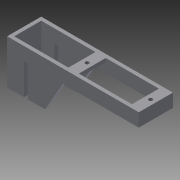
# Autodesk Inventor part: CarCab
Saved by Autodesk Inventor 2015 (Build 190159000, 159)
## iProperties
Created: 2016-04-06
Part Number: CarCab
Material: Generic
Document SubType Name: Modeling
Designer: Lee
Density: 1 g/cm^3
Appearance: Default
Author: Lee
Autodesk Inventor part; units mm, degrees
ref_plane "YZ Plane" through (0, 0, 0) normal (1, 0, 0) x (0, 1, 0)
ref_plane "XZ Plane" through (0, 0, 0) normal (0, 1, 0) x (-1, 0, 0)
ref_plane "XY Plane" through (0, 0, 0) normal (0, 0, 1) x (1, 0, 0)
sketch "Sketch1" plane through (0, 0, 0) normal (0, 0, 1) x (1, 0, 0)
  line L0 (0, 0) -> (59.5, 0)
  line L1 (59.5, 0) -> (59.5, 15.4)
  line L2 (59.5, 15.4) -> (0, 15.4)
  line L3 (0, 15.4) -> (0, 0)
  line L4 (1.6, 13.8) -> (57.9, 13.8)
  line L5 (57.9, 13.8) -> (57.9, 1.6)
  line L6 (57.9, 1.6) -> (1.6, 1.6)
  line L7 (1.6, 1.6) -> (1.6, 13.8)
  dimension "d0" = 59.5
  dimension "d1" = 15.4
  dimension "d2" = 1.6
  constraints: 16 end point, 4 parallel, 2 perpendicular, 1 horizontal, 3 other
  measures "d0" distance of L1.end L2.end
  measures "d1" distance of L2.end L0.start
  measures "d2" distance between parallel lines of L2 L4
extrude "Extrusion1" add sketch "Sketch1" along normal blind 20
sketch "Sketch2" plane through (0, 0, 0) normal (0, -1, 0) x (1, 0, 0)
  line L0 (1.6, 0) -> (57.9, 0) projected
  line L1 (7.6, 0) -> (9.2, 0)
  line L2 (9.2, 0) -> (9.2, 14)
  line L3 (9.2, 14) -> (7.6, 14)
  line L4 (7.6, 14) -> (7.6, 0)
  line L5 (0, 0) -> (0, 20) projected
  dimension "d5" = 1.6
  dimension "d6" = 14
  dimension "d7" = 7.6
  constraints: 8 end point, 2 parallel, 1 horizontal, 1 perpendicular, 1 point on line
  measures "d5" distance of L2.end L3.end
  measures "d6" distance of L1.end L2.end
  measures "d7" distance between parallel lines of L5 L4
extrude "Extrusion2" cut sketch "Sketch2" against normal up to surface (15.4 mm away)
sketch "Sketch3" plane through (0, 0, 20) normal (0, -1, 0) x (1, 0, 0)
  line L0 (9.2, -6) -> (9.2, -20) projected
  line L1 (9.2, -20) -> (59.5, -20) projected
  line L2 (59.5, -20) -> (59.5, 0) projected
  line L3 (0, 0) -> (59.5, 0) projected
  line L4 (0, -20) -> (0, 0) projected
  line L5 (0, -20) -> (7.6, -20) projected
  line L6 (7.6, -20) -> (7.6, -6) projected
  line L7 (7.6, -6) -> (9.2, -6) projected
  line L8 (57.9, -20) -> (9.2, -20) projected
  line L9 (25.2, -20) -> (59.5, -20)
  line L10 (59.5, -20) -> (59.5, -6)
  line L11 (59.5, -6) -> (25.2, -6)
  line L12 (25.2, -6) -> (25.2, -20)
  dimension "d10" = 14
  dimension "d11" = 16
  constraints: 8 end point, 2 parallel, 2 point on line, 1 horizontal, 1 perpendicular
  measures "d10" distance of L11.end L9.start
  measures "d11" distance between parallel lines of L0 L12
extrude "Extrusion3" cut sketch "Sketch3" against normal up to surface (15.4 mm away) contours L12 L11 L2 L1
sketch "Sketch4" plane through (0, 0, 20) normal (0, -1, 0) x (1, 0, 0)
  line L0 (25.2, -6) -> (59.5, -6) projected
  line L1 (59.5, -6) -> (59.5, 0) projected
  line L2 (0, 0) -> (59.5, 0) projected
  line L3 (0, -20) -> (0, 0) projected
  line L4 (0, -20) -> (7.6, -20) projected
  line L5 (7.6, -20) -> (7.6, -6) projected
  line L6 (7.6, -6) -> (9.2, -6) projected
  line L7 (9.2, -6) -> (9.2, -20) projected
  line L8 (9.2, -20) -> (25.2, -20) projected
  line L9 (25.2, -20) -> (25.2, -6) projected
  line L10 (59.5, 0) -> (54.8, 0)
  line L11 (54.8, 0) -> (54.8, -1.6)
  line L12 (54.8, -1.6) -> (59.5, -1.6)
  line L13 (59.5, -1.6) -> (59.5, 0)
  line L14 (57.9, 0) -> (1.6, 0) projected
  line L15 (30.8, 0) -> (26.1, 0)
  line L16 (26.1, 0) -> (26.1, -1.6)
  line L17 (26.1, -1.6) -> (30.8, -1.6)
  line L18 (30.8, -1.6) -> (30.8, 0)
  dimension "d14" = 4.7
  dimension "d15" = 1.6
  dimension "d16" = 1.6
  dimension "d17" = 4.7
  dimension "d18" = 24
  constraints: 16 end point, 4 parallel, 2 horizontal, 2 perpendicular, 1 point on line
  measures "d14" distance of L11.end L12.end
  measures "d15" distance of L10.end L11.end
  measures "d16" distance of L15.end L16.end
  measures "d17" distance of L16.end L17.end
  measures "d18" distance between parallel lines of L11 L18
extrude "Extrusion4" add sketch "Sketch4" against normal up to next contours L12 L11 L2 L1 | L18 L17 L16 L2
sketch "Sketch6" plane through (0, 0, 20) normal (0, 0, 1) x (1, 0, 0)
  line L0 (0, 0) -> (59.5, 0) projected
  line L1 (59.5, 0) -> (59.5, 15.4) projected
  line L2 (59.5, 15.4) -> (0, 15.4) projected
  line L3 (0, 15.4) -> (0, 0) projected
  line L4 (26.1, 1.6) -> (26.1, 13.8) projected
  line L5 (26.1, 1.6) -> (1.6, 1.6) projected
  line L6 (1.6, 1.6) -> (1.6, 13.8) projected
  line L7 (1.6, 13.8) -> (26.1, 13.8) projected
  line L8 (54.8, 1.6) -> (30.8, 1.6) projected
  line L9 (30.8, 1.6) -> (30.8, 13.8) projected
  line L10 (30.8, 13.8) -> (54.8, 13.8) projected
  line L11 (54.8, 1.6) -> (54.8, 13.8) projected
  line L12 (26.1, 1.6) -> (30.8, 13.8)
  line L13 (30.8, 1.6) -> (26.1, 13.8)
  line L14 (54.8, 1.6) -> (59.5, 1.6)
  line L15 (59.5, 0) -> (59.5, 15.4) projected
  line L16 (54.8, 13.8) -> (59.5, 13.8)
  line L17 (54.8, 1.6) -> (59.5, 13.8)
  line L18 (54.8, 13.8) -> (59.5, 1.6)
  circle A0 centre (28.45, 7.7) radius 0.85
  circle A1 centre (57.15, 7.7) radius 0.85
  point P0 (0, 0)
  dimension "d24" = 1.7
  dimension "d25" = 1.7
  constraints: 12 end point, 2 centre point, 2 midpoint, 2 point on line
  measures "d24" diameter of A0
  measures "d25" diameter of A1
extrude "Extrusion5" cut sketch "Sketch6" against normal up to next contours A1 L17 L18 | L18 L17 A1 | L17 L18 A1 | A1 L18 L17 | A0 L12 L13 | L13 L12 A0 | L12 L13 A0 | L12 A0 L13
sketch "Sketch7" plane through (0, 0, 20) normal (0, -1, 0) x (1, 0, 0)
  line L0 (59.5, -6) -> (59.5, 0) projected
  line L1 (0, 0) -> (59.5, 0) projected
  line L2 (0, -20) -> (0, 0) projected
  line L3 (0, -20) -> (7.6, -20) projected
  line L4 (7.6, -20) -> (7.6, -6) projected
  line L5 (7.6, -6) -> (9.2, -6) projected
  line L6 (9.2, -6) -> (9.2, -20) projected
  line L7 (9.2, -20) -> (25.2, -20) projected
  line L8 (25.2, -20) -> (25.2, -6) projected
  line L9 (25.2, -6) -> (59.5, -6) projected
  line L10 (25.2, -6) -> (17.1171, -20)
  line L11 (9.2, -20) -> (25.2, -20) projected
  line L12 (25.2, -6) -> (41.3658, -6) construction
  line L13 (17.1171, -20) -> (25.2, -20)
  line L14 (25.2, -20) -> (25.2, -6)
  dimension "d28" = 120
  constraints: 8 end point, 1 equal length, 1 horizontal, 1 point on line
  measures "d28" angle of L10 L12
extrude "Extrusion6" cut sketch "Sketch7" against normal up to surface (15.4 mm away) contours L8 L7 L10
body "Solid1"
